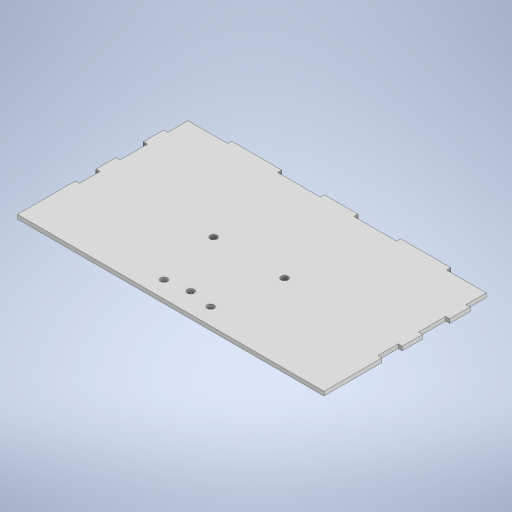
# Autodesk Inventor part: mieng_mat_3mm
Saved by Autodesk Inventor 2023 (Build 270158000, 158)
## iProperties
Created: 2022-11-20
Part Number: mieng_mat_3mm
Material: Generic
Document SubType Name: Modeling
Designer: ADMIN
Density: 1 g/cm^3
Appearance: Default
Author: ADMIN
Autodesk Inventor part; units mm, degrees
ref_plane "YZ Plane" through (0, 0, 0) normal (1, 0, 0) x (0, 1, 0)
ref_plane "XZ Plane" through (0, 0, 0) normal (0, 1, 0) x (-1, 0, 0)
ref_plane "XY Plane" through (0, 0, 0) normal (0, 0, 1) x (1, 0, 0)
sketch "Sketch1" plane through (0, 0, 0) normal (0, 1, 0) x (-1, 0, 0)
  line L0 (16.7044, 65.1664) -> (16.7044, 62.1664)
  line L1 (-20.3174, 65.1664) -> (-20.3174, 62.1664)
  line L2 (-51.677, 65.1664) -> (-51.677, 62.1664)
  line L3 (-144.9395, 65.1664) -> (-144.9395, 62.1664)
  line L4 (-107.9177, 65.1664) -> (-107.9177, 62.1664)
  line L5 (-76.5581, 65.1664) -> (-76.5581, 62.1664)
  line L6 (45.8824, 65.1664) -> (16.7044, 65.1664)
  line L7 (-64.1176, 62.1664) -> (-51.677, 62.1664)
  line L8 (-20.3174, 62.1664) -> (16.7044, 62.1664)
  line L9 (16.7044, 62.1664) -> (-20.3174, 62.1664)
  line L10 (-20.3174, 65.1664) -> (-51.677, 65.1664)
  line L11 (-51.677, 62.1664) -> (-76.5581, 62.1664)
  line L12 (-107.9177, 62.1664) -> (-144.9395, 62.1664)
  line L13 (-64.1176, 62.1664) -> (-76.5581, 62.1664)
  line L14 (-76.5581, 65.1664) -> (-107.9177, 65.1664)
  line L15 (-144.9395, 65.1664) -> (-174.1176, 65.1664)
  line L16 (48.8824, 80.1664) -> (48.8824, 95.1664)
  line L17 (48.8824, 95.1664) -> (45.8824, 95.1664)
  line L18 (48.8824, 80.1664) -> (45.8824, 80.1664)
  line L19 (48.8824, 115.1664) -> (45.8824, 115.1664)
  line L20 (48.8824, 130.1664) -> (45.8824, 130.1664)
  line L21 (-177.1176, 130.1664) -> (-174.1176, 130.1664)
  line L22 (-177.1176, 115.1664) -> (-174.1176, 115.1664)
  line L23 (-177.1176, 95.1664) -> (-174.1176, 95.1664)
  line L24 (-177.1176, 80.1664) -> (-174.1176, 80.1664)
  line L25 (45.8824, 80.1664) -> (45.8824, 65.1664)
  line L26 (48.8824, 115.1664) -> (48.8824, 130.1664)
  line L27 (45.8824, 145.1664) -> (45.8824, 130.1664)
  line L28 (45.8824, 115.1664) -> (45.8824, 95.1664)
  line L29 (-174.1176, 65.1664) -> (-174.1176, 80.1664)
  line L30 (-174.1176, 95.1664) -> (-174.1176, 115.1664)
  line L31 (-174.1176, 130.1664) -> (-174.1176, 145.1664)
  line L32 (-177.1176, 80.1664) -> (-177.1176, 95.1664)
  line L33 (-177.1176, 115.1664) -> (-177.1176, 130.1664)
  line L34 (-213.0378, 187.8664) -> (84.2595, 187.8664)
  line L35 (-177.1176, 187.8664) -> (-177.1176, 145.1664)
  line L36 (-177.1176, 145.1664) -> (-174.1176, 145.1664)
  line L37 (48.8824, 187.8664) -> (48.8824, 145.1664)
  line L38 (48.8824, 145.1664) -> (45.8824, 145.1664)
  circle A0 centre (-81.336, 175.651) radius 2.5
  circle A1 centre (-90.2887, 130.1664) radius 2.5
  circle A2 centre (-64.1176, 173.151) radius 2.5
  circle A3 centre (-46.8991, 175.651) radius 2.5
  circle A4 centre (-37.9465, 130.1664) radius 2.5
  point P0 (0, 0)
  point P1 (48.8824, 62.1664)
  point P2 (-126.4286, 62.1664)
  point P3 (-161.0285, 65.1664)
  point P4 (-177.1176, 122.6664)
  point P5 (48.8824, 122.6664)
  point P6 (-76.5581, 63.6664)
  point P7 (-51.677, 63.6664)
  dimension "d1" = 15
  dimension "d3" = 220
  dimension "d4" = 226
  dimension "d5" = 20
  dimension "d6" = 15
  dimension "d7" = 15
  dimension "d9" = 15
  dimension "d10" = 29.178
  dimension "d11" = 37.0218
  dimension "d12" = 31.3596
  dimension "d13" = 24.8811
  dimension "d14" = 31.3596
  dimension "d16" = 37.0218
  dimension "d17" = 29.178
  dimension "d18" = 15
  dimension "d19" = 15
  dimension "d20" = 20
  dimension "d21" = 15
  dimension "d22" = 15
  dimension "d23" = 3
  dimension "d24" = 3
  dimension "d27" = 122.7
  dimension "d28" = 5
  dimension "d29" = 5
  dimension "d30" = 65
  dimension "d31" = 5
  constraints: 78 end point, 25 perpendicular, 12 parallel, 11 horizontal, 5 centre point, 5 midpoint, 4 point on line, 2 vertical
  measures "d1" distance of L18.start L16.end
  measures "d3" distance of L31.end L27.start
  measures "d4" distance of point (-177.118, 122.666) point (48.882, 122.666)
  measures "d5" distance of L28.start L17.end
  measures "d6" distance of L19.start L26.end
  measures "d7" distance of L27.start L20.end
  measures "d9" distance of L25.start L25.end
  measures "d10" distance of L25.end L6.end
  measures "d11" distance of L8.start L0.end
  measures "d12" distance of L10.start L2.start
  measures "d13" distance of point (-76.558, 63.666) point (-51.677, 63.666)
  measures "d14" distance of L14.start L4.start
  measures "d16" distance of L4.end L3.end
  measures "d17" distance of L15.start L15.end
  measures "d18" distance of L15.end L29.end
  measures "d19" distance of L24.start L32.end
  measures "d20" distance of L30.start L30.end
  measures "d21" distance of L22.start L21.start
  measures "d22" distance of L21.end L31.end
  measures "d23" distance of L16.end L17.end
  measures "d24" distance of L6.end L0.end
  measures "d27" distance between parallel lines of L34 L15
  measures "d28" diameter of A0
  measures "d29" diameter of A1
  measures "d30" distance from line of L14 A1.centre
  measures "d31" diameter of A2
extrude "Extrusion1" add sketch "Sketch1" along normal blind 3
body "Solid1"
